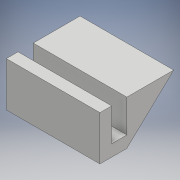
# Autodesk Inventor part: Ooze_Ramp_Bottom
Saved by Autodesk Inventor 2017 (Build 210142000, 142)
## iProperties
Created: 2017-01-16
Part Number: Ooze_Ramp_Bottom
Material: Generic
Document SubType Name: Modeling
Designer: willt
Density: 1 g/cm^3
Appearance: Default
Author: willt
Autodesk Inventor part; units mm, degrees
ref_plane "YZ Plane" through (0, 0, 0) normal (1, 0, 0) x (0, 1, 0)
ref_plane "XZ Plane" through (0, 0, 0) normal (0, 1, 0) x (-1, 0, 0)
ref_plane "XY Plane" through (0, 0, 0) normal (0, 0, 1) x (1, 0, 0)
sketch "Sketch1" plane through (0, 0, 0) normal (1, 0, 0) x (0, 1, 0)
  line L0 (0, 0) -> (20, 0)
  line L1 (20, 0) -> (0, -19)
  line L2 (0, -19) -> (0, 0)
  dimension "d0" = 20
  dimension "d1" = 19
  constraints: 6 end point, 1 horizontal, 1 perpendicular
  measures "d0" distance of L0.start L0.end
  measures "d1" distance of L1.end L0.start
extrude "Extrusion1" add sketch "Sketch1" along normal blind 40
sketch "Sketch2" plane through (0, 0, -19) normal (0, -1, 0) x (1, 0, 0)
  line L0 (40, 19) -> (40, 0) projected
  line L1 (40, 0) -> (0, 0)
  line L2 (0, 0) -> (0, 5)
  line L3 (0, 5) -> (40, 5)
  line L4 (40, 5) -> (40, 0)
  point P0 (0, 19)
  dimension "d4" = 5
  constraints: 8 end point, 2 parallel, 1 horizontal, 1 perpendicular
  measures "d4" distance of L1.end L2.end
extrude "Extrusion2" add sketch "Sketch2" along normal blind 11.5
sketch "Sketch3" plane through (0, 0, -14) normal (0, 0, 1) x (1, 0, 0)
  line L0 (40, 0) -> (40, -11.5) projected
  line L1 (0, -11.5) -> (40, -11.5)
  line L2 (40, -11.5) -> (40, -6.5)
  line L3 (40, -6.5) -> (0, -6.5)
  line L4 (0, -6.5) -> (0, -11.5)
  point P0 (0, 0)
  dimension "d7" = 5
  constraints: 8 end point, 2 parallel, 1 horizontal, 1 perpendicular, 1 point on line
  measures "d7" distance of L2.end L1.end
extrude "Extrusion3" add sketch "Sketch3" along normal blind 14
body "Solid1"
